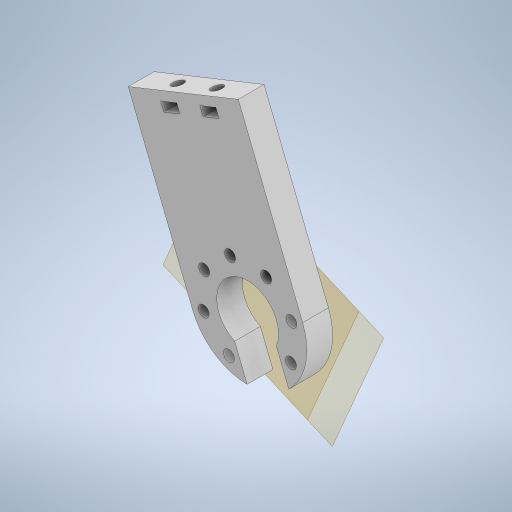
# Autodesk Inventor part: _foot_adt
Saved by Autodesk Inventor 2024.3 (Build 283343000, 343)
## iProperties
Created: 2024-09-06
Part Number: _foot_adt
Material: 일반
Document SubType Name: Modeling
Designer: gretc
Density: 1 g/cm^3
Appearance: 기본값
Author: gretc
Autodesk Inventor part; units mm, degrees
ref_plane "YZ Plane" through (0, 0, 0) normal (1, 0, 0) x (0, 1, 0)
ref_plane "XZ Plane" through (0, 0, 0) normal (0, 1, 0) x (-1, 0, 0)
ref_plane "XY Plane" through (0, 0, 0) normal (0, 0, 1) x (1, 0, 0)
ref_plane "작업 평면1" through (0, 0, 0) normal (0, 0, 1) x (0.3947, 0.9188, 0)
sketch "스케치1" plane through (0, 0, 0) normal (0, 0, 1) x (0.3947, 0.9188, 0)
  point P0 (0, 0)
ref_plane "작업 평면2" through (0, 0, 0) normal (0, 0, 1) x (0.3947, 0.9188, 0)
sketch "스케치2" plane through (0, 0, 0) normal (0, 0, 1) x (0.3947, 0.9188, 0)
  circle A0 centre (0, 0) radius 13.8 projected
  circle A1 centre (0, 0) radius 7.2 projected
  circle A2 centre (0, -11) radius 1.2812 projected
  circle A3 centre (-7.7782, -7.7782) radius 1.2812 projected
  circle A4 centre (-11, 0) radius 1.2812 projected
  circle A5 centre (-7.7782, 7.7782) radius 1.2812 projected
  circle A6 centre (0, 11) radius 1.2812 projected
  circle A7 centre (7.7782, 7.7782) radius 1.2812 projected
  circle A8 centre (11, 0) radius 1.2812 projected
  circle A9 centre (7.7782, -7.7782) radius 1.2812 projected
  line L0 (33.63, -33.63) -> (-32.0037, 32.0037)
  circle A10 centre (0, 0) radius 4.75 projected
  circle A11 centre (0, 0) radius 5.2245
  line L1 (3.6943, -3.6943) -> (-3.6943, 3.6943)
  line L2 (-3.6943, 3.6943) -> (-13.4523, -6.0637)
  line L3 (-13.4523, -6.0637) -> (-6.0637, -13.4523)
  line L4 (-6.0637, -13.4523) -> (3.6943, -3.6943)
  line L5 (9.7581, -9.7581) -> (-9.7581, 9.7581)
  line L6 (-9.7581, 9.7581) -> (18.8336, 38.3497)
  line L7 (18.8336, 38.3497) -> (38.3497, 18.8336)
  line L8 (38.3497, 18.8336) -> (9.7581, -9.7581)
  point P0 (0, 0)
  point P1 (-12.726, -5.3374)
  point P2 (-7.1975, 0.1912)
  point P3 (0.1912, -7.1975)
  point P4 (-5.3374, -12.726)
  constraints: 18 end point, 4 parallel, 4 point on circle, 4 point on line, 2 perpendicular, 1 centre point, 1 coincident, 1 collinear, 3 other
extrude "돌출1" add sketch "스케치2" along normal blind 6 contours A0 L0 A9 A1 A5 | A0 L6 L7 L8 | L0 A5 A1 L2 A0 | A0 L4 A1 L0 A9
sketch "스케치3" plane through (-27.8029, 32.4408, 6) normal (-0.3706, 0.9288, 0) x (0.9288, 0.3706, 0)
  line L0 (27.6, 6) -> (27.6, 0) projected
  line L1 (27.6, 6) -> (18.4, 6)
  line L2 (21, 6) -> (6.6, 6) projected
  line L3 (18.4, 6) -> (9.2, 6)
  line L4 (19.0245, 6) -> (19.0245, 3)
  line L5 (19.0245, 6) -> (19.0245, 0) projected
  line L6 (9.2, 6) -> (9.2, 3)
  circle A0 centre (19.0245, 3) radius 1.35
  circle A1 centre (9.2, 3) radius 1.35
  point P0 (13.8, 6)
  point P1 (8.5755, 6)
  dimension "d2" = 9.2
  dimension "d3" = 9.2
  dimension "d4" = 3
  dimension "d5" = 3
  dimension "d6" = 2.7
  dimension "d7" = 2.7
  constraints: 8 end point, 2 centre point, 2 coincident, 2 point on line, 1 midpoint, 1 vertical
  measures "d2" distance of L0.start L1.end
  measures "d3" distance of L1.end L3.end
  measures "d4" distance of L4.start L4.end
  measures "d5" distance of L3.end L6.end
  measures "d6" diameter of A0
  measures "d7" diameter of A1
extrude "돌출2" cut sketch "스케치3" against normal blind 3
sketch "스케치4" plane through (0, 0, 6) normal (0, 0, 1) x (0.9188, -0.3947, 0)
  line L0 (-23.7306, 29.2101) -> (-21.8214, 31.1192) projected
  line L1 (-30.6776, 22.2631) -> (-28.7684, 24.1722) projected
  line L2 (-23.7306, 29.2101) -> (-22.67, 30.2707)
  line L3 (-24.7913, 29.5636) -> (-21.9629, 32.392)
  line L4 (-21.9629, 32.392) -> (-20.5486, 30.9778)
  line L5 (-20.5486, 30.9778) -> (-23.3771, 28.1494)
  line L6 (-23.3771, 28.1494) -> (-24.7913, 29.5636)
  line L7 (-24.7913, 29.5636) -> (-20.5486, 30.9778) construction
  line L8 (-21.9629, 32.392) -> (-23.3771, 28.1494) construction
  line L9 (-30.6776, 22.2631) -> (-29.617, 23.3237)
  line L10 (-31.7383, 22.6166) -> (-28.9099, 25.445)
  line L11 (-28.9099, 25.445) -> (-27.4956, 24.0308)
  line L12 (-27.4956, 24.0308) -> (-30.3241, 21.2024)
  line L13 (-30.3241, 21.2024) -> (-31.7383, 22.6166)
  line L14 (-31.7383, 22.6166) -> (-27.4956, 24.0308) construction
  line L15 (-28.9099, 25.445) -> (-30.3241, 21.2024) construction
  point P0 (0, 0)
  dimension "d10" = 1.5
  dimension "d11" = 4
  dimension "d12" = 2
  dimension "d13" = 1.5
  dimension "d14" = 4
  constraints: 28 end point, 4 midpoint, 4 parallel, 2 perpendicular, 2 point on line
  measures "d10" distance of L0.start L2.end
  measures "d11" distance of L3.start L3.end
  measures "d12" distance of L3.end L4.end
  measures "d13" distance of L1.start L9.end
  measures "d14" distance of L10.start L10.end
extrude "돌출3" cut sketch "스케치4" against normal blind 3
sketch "스케치5" plane through (0, 0, 0) normal (0, 0, -1) x (-0.9188, 0.3947, 0)
  line L0 (21.8214, 31.1192) -> (23.7306, 29.2101) projected
  line L1 (28.7684, 24.1722) -> (30.6776, 22.2631) projected
  line L2 (21.8214, 31.1192) -> (22.8821, 30.0586)
  line L3 (28.7684, 24.1722) -> (29.8291, 23.1116)
  line L4 (23.5892, 27.9373) -> (25.0034, 29.3515)
  line L5 (25.0034, 29.3515) -> (22.175, 32.1799)
  line L6 (22.175, 32.1799) -> (20.7608, 30.7657)
  line L7 (20.7608, 30.7657) -> (23.5892, 27.9373)
  line L8 (23.5892, 27.9373) -> (22.175, 32.1799) construction
  line L9 (25.0034, 29.3515) -> (20.7608, 30.7657) construction
  line L10 (30.5362, 20.9903) -> (31.9504, 22.4045)
  line L11 (31.9504, 22.4045) -> (29.122, 25.2329)
  line L12 (29.122, 25.2329) -> (27.7078, 23.8187)
  line L13 (27.7078, 23.8187) -> (30.5362, 20.9903)
  line L14 (30.5362, 20.9903) -> (29.122, 25.2329) construction
  line L15 (31.9504, 22.4045) -> (27.7078, 23.8187) construction
  point P0 (0, 0)
  dimension "d17" = 1.5
  dimension "d18" = 1.5
  dimension "d19" = 2
  dimension "d20" = 4
  dimension "d21" = 4
  constraints: 28 end point, 4 midpoint, 4 parallel, 4 perpendicular, 2 point on line
  measures "d17" distance of L0.start L2.end
  measures "d18" distance of L1.start L3.end
  measures "d19" distance of L4.start L4.end
  measures "d20" distance of L5.end L4.end
  measures "d21" distance of L11.end L10.end
extrude "돌출4" cut sketch "스케치5" against normal blind 3
